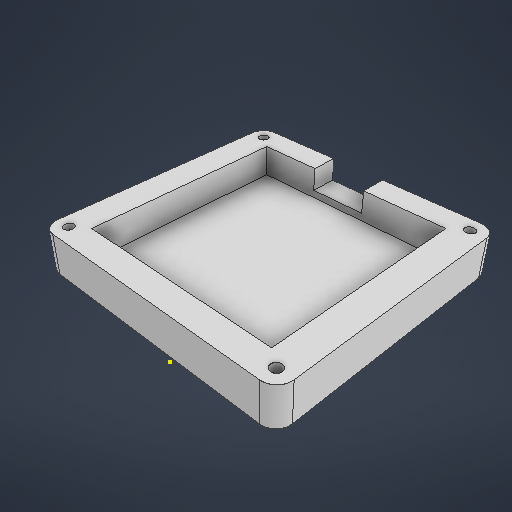
# Autodesk Inventor part: Case_Bottom
Saved by Autodesk Inventor 2026.1 (Build 301233000, 233)
## iProperties
Created: 2025-12-06
Part Number: Case_Bottom
Material: Generic
Document SubType Name: Modeling
Designer: chest
Density: 1 g/cm^3
Appearance: Default
Author: chest
Autodesk Inventor part; units mm, degrees
ref_plane "YZ Plane" through (0, 0, 0) normal (1, 0, 0) x (0, 1, 0)
ref_plane "XZ Plane" through (0, 0, 0) normal (0, 1, 0) x (-1, 0, 0)
ref_plane "XY Plane" through (0, 0, 0) normal (0, 0, 1) x (1, 0, 0)
sketch "Sketch1" plane through (0, 0, 0) normal (0, 1, 0) x (-1, 0, 0)
  line L0 (54.6183, -19.0153) -> (-12.4217, -19.0153)
  line L1 (-12.4217, -19.0153) -> (-12.4217, -83.5153)
  line L2 (-12.4217, -83.5153) -> (54.6183, -83.5153)
  line L3 (54.6183, -83.5153) -> (54.6183, -19.0153)
  line L4 (-21.9217, -9.5153) -> (64.1183, -9.5153)
  line L5 (64.1183, -9.5153) -> (64.1183, -93.0153)
  line L6 (64.1183, -93.0153) -> (-21.9217, -93.0153)
  line L7 (-21.9217, -93.0153) -> (-21.9217, -9.5153)
  circle A0 centre (-16.9217, -14.5153) radius 1.7
  circle A1 centre (-16.9217, -88.0153) radius 1.7
  circle A2 centre (59.1183, -88.0153) radius 1.7
  circle A3 centre (59.1183, -14.5153) radius 1.7
  circle A4 centre (59.1183, -14.5153) radius 3
  circle A5 centre (-16.9217, -14.5153) radius 3
  circle A6 centre (-16.9217, -88.0153) radius 3
  circle A7 centre (59.1183, -88.0153) radius 3
  point P0 (0, 0)
  point P1 (64.1183, -51.2653)
  dimension "d0" = 67.04
  dimension "d1" = 64.5
  dimension "d2" = 86.04
  dimension "d3" = 83.5
  dimension "d4" = 9.5
  dimension "d5" = 9.5
  dimension "d6" = 3.4
  dimension "d7" = 5
  dimension "d8" = 5
  dimension "d9" = 3.4
  dimension "d10" = 5
  dimension "d11" = 5
  dimension "d12" = 3.4
  dimension "d13" = 5
  dimension "d14" = 5
  dimension "d15" = 3.4
  dimension "d16" = 5
  dimension "d17" = 5
  dimension "d18" = 6
  dimension "d19" = 6
  dimension "d20" = 6
  dimension "d21" = 6
  constraints: 16 end point, 8 centre point, 4 coincident, 4 parallel, 2 horizontal, 2 perpendicular, 1 midpoint
  measures "d0" distance of L2.end L1.end
  measures "d1" distance of L1.end L0.end
  measures "d2" distance of L5.end L6.end
  measures "d3" distance of L4.end L5.end
  measures "d4" distance between parallel lines of L6 L2
  measures "d5" distance from line of point (64.118, -51.265) L3
  measures "d6" diameter of A0
  measures "d7" distance from line of L4 A0.centre
  measures "d8" distance from line of L7 A0.centre
  measures "d9" diameter of A1
  measures "d10" distance from line of L7 A1.centre
  measures "d11" distance from line of L6 A1.centre
  measures "d12" diameter of A2
  measures "d13" distance from line of L6 A2.centre
  measures "d14" distance from line of L5 A2.centre
  measures "d15" diameter of A3
  measures "d16" distance from line of L5 A3.centre
  measures "d17" distance from line of L4 A3.centre
  measures "d18" diameter of A4
  measures "d19" diameter of A5
  measures "d20" diameter of A6
  measures "d21" diameter of A7
extrude "Extrusion1" add sketch "Sketch1" along normal blind 13 contours L3 L2 L1 L0 | L4 L5 L6 L7 | A0 | A1 | A2 | A3 | A4 | A5 | A6 | A7
sketch "Sketch3" plane through (0, 13, 0) normal (0, 1, 0) x (1, 0, 0)
  circle A0 centre (-59.1183, 14.5153) radius 1.7
  line L0 (-64.1183, 9.5153) -> (21.9217, 9.5153) projected
  line L1 (-64.1183, 93.0153) -> (-64.1183, 9.5153) projected
  circle A1 centre (16.9217, 14.5153) radius 1.7
  line L2 (21.9217, 9.5153) -> (21.9217, 93.0153) projected
  circle A2 centre (16.9217, 88.0153) radius 1.7
  line L3 (21.9217, 93.0153) -> (-64.1183, 93.0153) projected
  circle A3 centre (-59.1183, 88.0153) radius 1.7
  point P0 (0, 0)
  dimension "d24" = 3.4
  dimension "d25" = 5
  dimension "d26" = 5
  dimension "d27" = 3.4
  dimension "d28" = 5
  dimension "d29" = 5
  dimension "d30" = 3.4
  dimension "d31" = 5
  dimension "d32" = 5
  dimension "d33" = 3.4
  dimension "d34" = 5
  dimension "d35" = 5
  constraints: 4 centre point
  measures "d24" diameter of A0
  measures "d25" distance from line of L0 A0.centre
  measures "d26" distance from line of A0.centre L1
  measures "d27" diameter of A1
  measures "d28" distance from line of L0 A1.centre
  measures "d29" distance from line of L2 A1.centre
  measures "d30" diameter of A2
  measures "d31" distance from line of L3 A2.centre
  measures "d32" distance from line of L2 A2.centre
  measures "d33" diameter of A3
  measures "d34" distance from line of L3 A3.centre
  measures "d35" distance from line of L1 A3.centre
extrude "Extrusion2" cut sketch "Sketch3" against normal blind 13 contours A0 | A1 | A2 | A3
sketch "Sketch6" plane through (0, 13, 0) normal (0, 1, 0) x (1, 0, 0)
  point P0 (0, 0)
sketch "Sketch7" plane through (0, 13, 0) normal (0, 1, 0) x (1, 0, 0)
  line L0 (21.9217, 93.0153) -> (-64.1183, 93.0153) projected
  line L1 (-54.1183, 84.2853) -> (11.9217, 84.2853)
  line L2 (21.9217, 9.5153) -> (21.9217, 93.0153) projected
  line L3 (-64.1183, 9.5153) -> (21.9217, 9.5153) projected
  line L4 (-21.0983, 18.2453) -> (-54.1183, 18.2453)
  line L5 (-21.0983, 18.2453) -> (11.9217, 18.2453)
  line L6 (-54.1183, 84.2853) -> (-54.1183, 18.2453)
  line L7 (11.9217, 18.2453) -> (11.9217, 84.2853)
  point P0 (0, 0)
  constraints: 10 end point, 1 parallel, 1 vertical
extrude "Extrusion3" cut sketch "Sketch7" against normal blind 10
fillet "Fillet1" radius 5 4 edges at (-64.1183, 6.5, -9.5153) (21.9217, 6.5, -9.5153) (21.9217, 6.5, -93.0153) (-64.1183, 6.5, -93.0153)
sketch "Sketch8" plane through (0, 13, 0) normal (0, 1, 0) x (1, 0, 0)
  line L0 (-54.1183, 84.2853) -> (11.9217, 84.2853) projected
  line L1 (16.9217, 93.0153) -> (-59.1183, 93.0153) projected
  line L2 (-34.1183, 84.2853) -> (-15.6183, 84.2853)
  line L3 (-15.6183, 84.2853) -> (-15.6183, 93.0153)
  line L4 (-15.6183, 93.0153) -> (-34.1183, 93.0153)
  line L5 (-34.1183, 93.0153) -> (-34.1183, 84.2853)
  line L6 (-64.1183, 88.0153) -> (-64.1183, 14.5153) projected
  point P0 (0, 0)
  dimension "d48" = 18.5
  dimension "d49" = 30
  constraints: 8 end point, 2 parallel, 2 point on line, 1 horizontal, 1 perpendicular
  measures "d48" distance of L4.end L3.end
  measures "d49" distance between parallel lines of L6 L5
extrude "Extrusion4" cut sketch "Sketch8" against normal blind 7.5
sketch "Sketch9" plane through (0, 0, 0) normal (0, -1, 0) x (1, 0, 0)
  line L0 (11.89, -89.9498) -> (-24.6442, -89.9498) construction
  line L1 (-24.6442, -89.9498) -> (-24.6442, -85.133) construction
  line L2 (-24.6442, -85.133) -> (11.89, -85.133) construction
  line L3 (11.89, -85.133) -> (11.89, -89.9498) construction
  spline S0 degree 2 poles (9.1235, -86.3163) (9.4199, -86.3163) (9.9213, -86.5164) (10.1041, -86.7164) knots 0 0 0 1 2 2 2
  spline S1 degree 2 poles (10.1041, -86.7164) (10.2869, -86.914) (10.4869, -87.5068) (10.4869, -87.8922) knots 0 0 0 1 2 2 2
  spline S2 degree 2 poles (10.4869, -87.8922) (10.4869, -88.275) (10.2918, -88.8431) (10.1066, -89.0531) knots 0 0 0 1 2 2 2
  spline S3 degree 2 poles (10.1066, -89.0531) (9.9238, -89.2581) (9.4248, -89.473) (9.1161, -89.473) knots 0 0 0 1 2 2 2
  spline S4 degree 2 poles (9.1161, -89.473) (8.9629, -89.473) (8.6937, -89.4285) (8.5801, -89.3939) knots 0 0 0 1 2 2 2
  spline S5 degree 2 poles (8.5801, -89.3939) (8.4813, -89.3618) (8.2763, -89.2704) (8.175, -89.2161) knots 0 0 0 1 2 2 2
  line L4 (8.175, -89.2161) -> (8.175, -88.727)
  line L5 (8.175, -88.727) -> (8.2071, -88.727)
  spline S6 degree 2 poles (8.2071, -88.727) (8.2615, -88.7764) (8.4294, -88.9147) (8.5504, -88.9814) knots 0 0 0 1 2 2 2
  spline S7 degree 2 poles (8.5504, -88.9814) (8.6665, -89.0457) (8.9407, -89.1272) (9.1186, -89.1272) knots 0 0 0 1 2 2 2
  spline S8 degree 2 poles (9.1186, -89.1272) (9.3137, -89.1272) (9.662, -88.9666) (9.7929, -88.8135) knots 0 0 0 1 2 2 2
  spline S9 degree 2 poles (9.7929, -88.8135) (9.9213, -88.6579) (10.0646, -88.1861) (10.0646, -87.8922) knots 0 0 0 1 2 2 2
  spline S10 degree 2 poles (10.0646, -87.8922) (10.0646, -87.5785) (9.9139, -87.1265) (9.783, -86.9708) knots 0 0 0 1 2 2 2
  spline S11 degree 2 poles (9.783, -86.9708) (9.6545, -86.8202) (9.3112, -86.667) (9.1186, -86.667) knots 0 0 0 1 2 2 2
  spline S12 degree 2 poles (9.1186, -86.667) (8.9432, -86.667) (8.6443, -86.7535) (8.5282, -86.8177) knots 0 0 0 1 2 2 2
  spline S13 degree 2 poles (8.5282, -86.8177) (8.4171, -86.8819) (8.2516, -87.0153) (8.2046, -87.0622) knots 0 0 0 1 2 2 2
  line L6 (8.2046, -87.0622) -> (8.175, -87.0622)
  line L7 (8.175, -87.0622) -> (8.175, -86.5781)
  spline S14 degree 2 poles (8.175, -86.5781) (8.2763, -86.5312) (8.4541, -86.4447) (8.5801, -86.4052) knots 0 0 0 1 2 2 2
  spline S15 degree 2 poles (8.5801, -86.4052) (8.7135, -86.3608) (8.9407, -86.3163) (9.1235, -86.3163) knots 0 0 0 1 2 2 2
  line L8 (6.031, -86.3706) -> (6.4164, -86.3706)
  line L9 (6.4164, -86.3706) -> (6.4164, -87.6748)
  spline S16 degree 2 poles (6.4164, -87.6748) (6.4164, -87.8329) (6.446, -88.1046) (6.4905, -88.1861) knots 0 0 0 1 2 2 2
  spline S17 degree 2 poles (6.4905, -88.1861) (6.5374, -88.2725) (6.7053, -88.3565) (6.8486, -88.3565) knots 0 0 0 1 2 2 2
  spline S18 degree 2 poles (6.8486, -88.3565) (6.9919, -88.3565) (7.2957, -88.2034) (7.4414, -88.0799) knots 0 0 0 1 2 2 2
  line L10 (7.4414, -88.0799) -> (7.4414, -86.3706)
  line L11 (7.4414, -86.3706) -> (7.8267, -86.3706)
  line L12 (7.8267, -86.3706) -> (7.8267, -89.5545)
  line L13 (7.8267, -89.5545) -> (7.4414, -89.5545)
  line L14 (7.4414, -89.5545) -> (7.4414, -88.4035)
  spline S19 degree 2 poles (7.4414, -88.4035) (7.2685, -88.5591) (6.9351, -88.7221) (6.7473, -88.7221) knots 0 0 0 1 2 2 2
  spline S20 degree 2 poles (6.7473, -88.7221) (6.4114, -88.7221) (6.031, -88.2775) (6.031, -87.8551) knots 0 0 0 1 2 2 2
  line L15 (6.031, -87.8551) -> (6.031, -86.3706)
  spline S21 degree 2 poles (4.4971, -86.3188) (5.0455, -86.3188) (5.6482, -86.9338) (5.6482, -87.5019) knots 0 0 0 1 2 2 2
  spline S22 degree 2 poles (5.6482, -87.5019) (5.6482, -88.0601) (5.0628, -88.7221) (4.591, -88.7221) knots 0 0 0 1 2 2 2
  spline S23 degree 2 poles (4.591, -88.7221) (4.3786, -88.7221) (4.0501, -88.5986) (3.929, -88.4677) knots 0 0 0 1 2 2 2
  spline S24 degree 2 poles (3.929, -88.4677) (3.8055, -88.3368) (3.6746, -87.9589) (3.6746, -87.6847) knots 0 0 0 1 2 2 2
  line L16 (3.6746, -87.6847) -> (3.6746, -87.4747)
  line L17 (3.6746, -87.4747) -> (5.2579, -87.4747)
  spline S25 degree 2 poles (5.2579, -87.4747) (5.2579, -87.0771) (4.8578, -86.6547) (4.5021, -86.6547) knots 0 0 0 1 2 2 2
  spline S26 degree 2 poles (4.5021, -86.6547) (4.3761, -86.6547) (4.1316, -86.7115) (4.0328, -86.756) knots 0 0 0 1 2 2 2
  spline S27 degree 2 poles (4.0328, -86.756) (3.929, -86.8054) (3.7858, -86.8918) (3.7389, -86.9313) knots 0 0 0 1 2 2 2
  line L18 (3.7389, -86.9313) -> (3.7166, -86.9313)
  line L19 (3.7166, -86.9313) -> (3.7166, -86.5114)
  spline S28 degree 2 poles (3.7166, -86.5114) (3.7833, -86.4843) (3.9859, -86.4052) (4.0649, -86.383) knots 0 0 0 1 2 2 2
  spline S29 degree 2 poles (4.0649, -86.383) (4.176, -86.3509) (4.3588, -86.3188) (4.4971, -86.3188) knots 0 0 0 1 2 2 2
  spline S30 degree 2 poles (4.0501, -87.7687) (4.055, -87.9243) (4.1192, -88.1515) (4.181, -88.2281) knots 0 0 0 1 2 2 2
  spline S31 degree 2 poles (4.181, -88.2281) (4.2477, -88.3145) (4.4576, -88.4059) (4.6132, -88.4059) knots 0 0 0 1 2 2 2
  spline S32 degree 2 poles (4.6132, -88.4059) (4.7664, -88.4059) (4.9813, -88.3145) (5.0702, -88.2256) knots 0 0 0 1 2 2 2
  spline S33 degree 2 poles (5.0702, -88.2256) (5.1566, -88.1342) (5.2456, -87.9144) (5.2579, -87.7687) knots 0 0 0 1 2 2 2
  line L20 (5.2579, -87.7687) -> (4.0501, -87.7687)
  spline S34 degree 2 poles (2.6669, -86.3163) (2.8966, -86.3163) (3.2943, -86.4398) (3.4252, -86.509) knots 0 0 0 1 2 2 2
  line L21 (3.4252, -86.509) -> (3.4252, -86.9412)
  line L22 (3.4252, -86.9412) -> (3.4054, -86.9412)
  spline S35 degree 2 poles (3.4054, -86.9412) (3.356, -86.9017) (3.2226, -86.8078) (3.1115, -86.756) knots 0 0 0 1 2 2 2
  spline S36 degree 2 poles (3.1115, -86.756) (3.0151, -86.709) (2.778, -86.6399) (2.652, -86.6399) knots 0 0 0 1 2 2 2
  spline S37 degree 2 poles (2.652, -86.6399) (2.5607, -86.6399) (2.3507, -86.6819) (2.3013, -86.7164) knots 0 0 0 1 2 2 2
  spline S38 degree 2 poles (2.3013, -86.7164) (2.2297, -86.7634) (2.1655, -86.8696) (2.1655, -86.9783) knots 0 0 0 1 2 2 2
  spline S39 degree 2 poles (2.1655, -86.9783) (2.1655, -87.1141) (2.3137, -87.2549) (2.5038, -87.3018) knots 0 0 0 1 2 2 2
  spline S40 degree 2 poles (2.5038, -87.3018) (2.5779, -87.3191) (2.8151, -87.3685) (2.9163, -87.3957) knots 0 0 0 1 2 2 2
  spline S41 degree 2 poles (2.9163, -87.3957) (3.1782, -87.4723) (3.4153, -87.7884) (3.4153, -88.0132) knots 0 0 0 1 2 2 2
  spline S42 degree 2 poles (3.4153, -88.0132) (3.4153, -88.3244) (2.9484, -88.7122) (2.5631, -88.7122) knots 0 0 0 1 2 2 2
  spline S43 degree 2 poles (2.5631, -88.7122) (2.3729, -88.7122) (1.9876, -88.6183) (1.8567, -88.5467) knots 0 0 0 1 2 2 2
  line L23 (1.8567, -88.5467) -> (1.8567, -88.1342)
  line L24 (1.8567, -88.1342) -> (1.8765, -88.1342)
  spline S44 degree 2 poles (1.8765, -88.1342) (2.0247, -88.2528) (2.3853, -88.3886) (2.5705, -88.3886) knots 0 0 0 1 2 2 2
  spline S45 degree 2 poles (2.5705, -88.3886) (2.7607, -88.3886) (3.0226, -88.2281) (3.0226, -88.0675) knots 0 0 0 1 2 2 2
  spline S46 degree 2 poles (3.0226, -88.0675) (3.0226, -87.9218) (2.8669, -87.781) (2.694, -87.7366) knots 0 0 0 1 2 2 2
  spline S47 degree 2 poles (2.694, -87.7366) (2.6101, -87.7143) (2.3976, -87.6699) (2.2815, -87.6427) knots 0 0 0 1 2 2 2
  spline S48 degree 2 poles (2.2815, -87.6427) (2.0296, -87.5785) (1.7727, -87.2845) (1.7727, -87.0301) knots 0 0 0 1 2 2 2
  spline S49 degree 2 poles (1.7727, -87.0301) (1.7727, -86.8819) (1.8888, -86.6201) (2.0024, -86.5238) knots 0 0 0 1 2 2 2
  spline S50 degree 2 poles (2.0024, -86.5238) (2.1235, -86.4225) (2.4322, -86.3163) (2.6669, -86.3163) knots 0 0 0 1 2 2 2
  spline S51 degree 2 poles (0.723, -86.3262) (1.0367, -86.3262) (1.3899, -86.6843) (1.3899, -87.0721) knots 0 0 0 1 2 2 2
  line L25 (1.3899, -87.0721) -> (1.3899, -88.3392)
  line L26 (1.3899, -88.3392) -> (1.6492, -88.3392)
  line L27 (1.6492, -88.3392) -> (1.6492, -88.6579)
  line L28 (1.6492, -88.6579) -> (1.3899, -88.6579)
  line L29 (1.3899, -88.6579) -> (1.3899, -89.3149)
  line L30 (1.3899, -89.3149) -> (1.0045, -89.3149)
  line L31 (1.0045, -89.3149) -> (1.0045, -88.6579)
  line L32 (1.0045, -88.6579) -> (0.2957, -88.6579)
  line L33 (0.2957, -88.6579) -> (0.2957, -88.3392)
  line L34 (0.2957, -88.3392) -> (1.0045, -88.3392)
  line L35 (1.0045, -88.3392) -> (1.0045, -87.25)
  spline S52 degree 2 poles (1.0045, -87.25) (1.0045, -87.0771) (0.9922, -86.8869) (0.9502, -86.8054) knots 0 0 0 1 2 2 2
  spline S53 degree 2 poles (0.9502, -86.8054) (0.9156, -86.7337) (0.76, -86.6621) (0.6266, -86.6621) knots 0 0 0 1 2 2 2
  spline S54 degree 2 poles (0.6266, -86.6621) (0.5328, -86.6621) (0.3574, -86.7189) (0.3179, -86.7362) knots 0 0 0 1 2 2 2
  line L36 (0.3179, -86.7362) -> (0.2957, -86.7362)
  line L37 (0.2957, -86.7362) -> (0.2957, -86.3904)
  spline S55 degree 2 poles (0.2957, -86.3904) (0.4043, -86.3608) (0.6266, -86.3262) (0.723, -86.3262) knots 0 0 0 1 2 2 2
  spline S56 degree 2 poles (-0.9813, -86.3188) (-0.433, -86.3188) (0.1697, -86.9338) (0.1697, -87.5019) knots 0 0 0 1 2 2 2
  spline S57 degree 2 poles (0.1697, -87.5019) (0.1697, -88.0601) (-0.4157, -88.7221) (-0.8875, -88.7221) knots 0 0 0 1 2 2 2
  spline S58 degree 2 poles (-0.8875, -88.7221) (-1.0999, -88.7221) (-1.4284, -88.5986) (-1.5494, -88.4677) knots 0 0 0 1 2 2 2
  spline S59 degree 2 poles (-1.5494, -88.4677) (-1.673, -88.3368) (-1.8039, -87.9589) (-1.8039, -87.6847) knots 0 0 0 1 2 2 2
  line L38 (-1.8039, -87.6847) -> (-1.8039, -87.4747)
  line L39 (-1.8039, -87.4747) -> (-0.2206, -87.4747)
  spline S60 degree 2 poles (-0.2206, -87.4747) (-0.2206, -87.0771) (-0.6207, -86.6547) (-0.9764, -86.6547) knots 0 0 0 1 2 2 2
  spline S61 degree 2 poles (-0.9764, -86.6547) (-1.1024, -86.6547) (-1.3469, -86.7115) (-1.4457, -86.756) knots 0 0 0 1 2 2 2
  spline S62 degree 2 poles (-1.4457, -86.756) (-1.5494, -86.8054) (-1.6927, -86.8918) (-1.7396, -86.9313) knots 0 0 0 1 2 2 2
  line L40 (-1.7396, -86.9313) -> (-1.7619, -86.9313)
  line L41 (-1.7619, -86.9313) -> (-1.7619, -86.5114)
  spline S63 degree 2 poles (-1.7619, -86.5114) (-1.6952, -86.4843) (-1.4926, -86.4052) (-1.4136, -86.383) knots 0 0 0 1 2 2 2
  spline S64 degree 2 poles (-1.4136, -86.383) (-1.3024, -86.3509) (-1.1197, -86.3188) (-0.9813, -86.3188) knots 0 0 0 1 2 2 2
  spline S65 degree 2 poles (-1.4284, -87.7687) (-1.4235, -87.9243) (-1.3593, -88.1515) (-1.2975, -88.2281) knots 0 0 0 1 2 2 2
  spline S66 degree 2 poles (-1.2975, -88.2281) (-1.2308, -88.3145) (-1.0209, -88.4059) (-0.8653, -88.4059) knots 0 0 0 1 2 2 2
  spline S67 degree 2 poles (-0.8653, -88.4059) (-0.7121, -88.4059) (-0.4972, -88.3145) (-0.4083, -88.2256) knots 0 0 0 1 2 2 2
  spline S68 degree 2 poles (-0.4083, -88.2256) (-0.3219, -88.1342) (-0.2329, -87.9144) (-0.2206, -87.7687) knots 0 0 0 1 2 2 2
  line L42 (-0.2206, -87.7687) -> (-1.4284, -87.7687)
  line L43 (-3.4069, -88.2454) -> (-3.3871, -88.2454)
  spline S69 degree 2 poles (-3.3871, -88.2454) (-3.3427, -88.2577) (-3.2464, -88.2627) (-3.1797, -88.2627) knots 0 0 0 1 2 2 2
  spline S70 degree 2 poles (-3.1797, -88.2627) (-3.024, -88.2627) (-2.7178, -88.1268) (-2.5794, -87.9934) knots 0 0 0 1 2 2 2
  line L44 (-2.5794, -87.9934) -> (-2.5794, -86.3706)
  line L45 (-2.5794, -86.3706) -> (-2.1941, -86.3706)
  line L46 (-2.1941, -86.3706) -> (-2.1941, -88.6579)
  line L47 (-2.1941, -88.6579) -> (-2.5794, -88.6579)
  line L48 (-2.5794, -88.6579) -> (-2.5794, -88.317)
  spline S71 degree 2 poles (-2.5794, -88.317) (-2.7894, -88.5047) (-3.1031, -88.6579) (-3.2513, -88.6579) knots 0 0 0 1 2 2 2
  spline S72 degree 2 poles (-3.2513, -88.6579) (-3.3106, -88.6579) (-3.3699, -88.6529) (-3.4069, -88.6455) knots 0 0 0 1 2 2 2
  line L49 (-3.4069, -88.6455) -> (-3.4069, -88.2454)
  line L50 (-4.096, -89.5545) -> (-4.0071, -88.3689)
  line L51 (-4.0071, -88.3689) -> (-3.7305, -88.3689)
  line L52 (-3.7305, -88.3689) -> (-3.6416, -89.5545)
  line L53 (-3.6416, -89.5545) -> (-4.096, -89.5545)
  spline S73 degree 2 poles (-5.2075, -86.3163) (-4.9778, -86.3163) (-4.5802, -86.4398) (-4.4492, -86.509) knots 0 0 0 1 2 2 2
  line L54 (-4.4492, -86.509) -> (-4.4492, -86.9412)
  line L55 (-4.4492, -86.9412) -> (-4.469, -86.9412)
  spline S74 degree 2 poles (-4.469, -86.9412) (-4.5184, -86.9017) (-4.6518, -86.8078) (-4.7629, -86.756) knots 0 0 0 1 2 2 2
  spline S75 degree 2 poles (-4.7629, -86.756) (-4.8593, -86.709) (-5.0964, -86.6399) (-5.2224, -86.6399) knots 0 0 0 1 2 2 2
  spline S76 degree 2 poles (-5.2224, -86.6399) (-5.3138, -86.6399) (-5.5237, -86.6819) (-5.5731, -86.7164) knots 0 0 0 1 2 2 2
  spline S77 degree 2 poles (-5.5731, -86.7164) (-5.6447, -86.7634) (-5.709, -86.8696) (-5.709, -86.9783) knots 0 0 0 1 2 2 2
  spline S78 degree 2 poles (-5.709, -86.9783) (-5.709, -87.1141) (-5.5608, -87.2549) (-5.3706, -87.3018) knots 0 0 0 1 2 2 2
  spline S79 degree 2 poles (-5.3706, -87.3018) (-5.2965, -87.3191) (-5.0593, -87.3685) (-4.9581, -87.3957) knots 0 0 0 1 2 2 2
  spline S80 degree 2 poles (-4.9581, -87.3957) (-4.6963, -87.4723) (-4.4591, -87.7884) (-4.4591, -88.0132) knots 0 0 0 1 2 2 2
  spline S81 degree 2 poles (-4.4591, -88.0132) (-4.4591, -88.3244) (-4.926, -88.7122) (-5.3113, -88.7122) knots 0 0 0 1 2 2 2
  spline S82 degree 2 poles (-5.3113, -88.7122) (-5.5015, -88.7122) (-5.8868, -88.6183) (-6.0177, -88.5467) knots 0 0 0 1 2 2 2
  line L56 (-6.0177, -88.5467) -> (-6.0177, -88.1342)
  line L57 (-6.0177, -88.1342) -> (-5.9979, -88.1342)
  spline S83 degree 2 poles (-5.9979, -88.1342) (-5.8497, -88.2528) (-5.4891, -88.3886) (-5.3039, -88.3886) knots 0 0 0 1 2 2 2
  spline S84 degree 2 poles (-5.3039, -88.3886) (-5.1137, -88.3886) (-4.8519, -88.2281) (-4.8519, -88.0675) knots 0 0 0 1 2 2 2
  spline S85 degree 2 poles (-4.8519, -88.0675) (-4.8519, -87.9218) (-5.0075, -87.781) (-5.1804, -87.7366) knots 0 0 0 1 2 2 2
  spline S86 degree 2 poles (-5.1804, -87.7366) (-5.2644, -87.7143) (-5.4768, -87.6699) (-5.5929, -87.6427) knots 0 0 0 1 2 2 2
  spline S87 degree 2 poles (-5.5929, -87.6427) (-5.8448, -87.5785) (-6.1017, -87.2845) (-6.1017, -87.0301) knots 0 0 0 1 2 2 2
  spline S88 degree 2 poles (-6.1017, -87.0301) (-6.1017, -86.8819) (-5.9856, -86.6201) (-5.872, -86.5238) knots 0 0 0 1 2 2 2
  spline S89 degree 2 poles (-5.872, -86.5238) (-5.7509, -86.4225) (-5.4422, -86.3163) (-5.2075, -86.3163) knots 0 0 0 1 2 2 2
  line L58 (-10.0117, -86.3706) -> (-9.6066, -86.3706)
  line L59 (-9.6066, -86.3706) -> (-9.6066, -87.8625)
  line L60 (-9.6066, -87.8625) -> (-8.2037, -87.8625)
  line L61 (-8.2037, -87.8625) -> (-8.2037, -86.3706)
  line L62 (-8.2037, -86.3706) -> (-7.7986, -86.3706)
  line L63 (-7.7986, -86.3706) -> (-7.7986, -89.4186)
  line L64 (-7.7986, -89.4186) -> (-8.2037, -89.4186)
  line L65 (-8.2037, -89.4186) -> (-8.2037, -88.2231)
  line L66 (-8.2037, -88.2231) -> (-9.6066, -88.2231)
  line L67 (-9.6066, -88.2231) -> (-9.6066, -89.4186)
  line L68 (-9.6066, -89.4186) -> (-10.0117, -89.4186)
  line L69 (-10.0117, -89.4186) -> (-10.0117, -86.3706)
  spline S90 degree 2 poles (-11.8741, -86.6127) (-11.8272, -86.5781) (-11.6691, -86.4546) (-11.595, -86.4176) knots 0 0 0 1 2 2 2
  spline S91 degree 2 poles (-11.595, -86.4176) (-11.4937, -86.3632) (-11.3035, -86.3064) (-11.1306, -86.3064) knots 0 0 0 1 2 2 2
  spline S92 degree 2 poles (-11.1306, -86.3064) (-10.9899, -86.3064) (-10.7354, -86.4126) (-10.6391, -86.509) knots 0 0 0 1 2 2 2
  spline S93 degree 2 poles (-10.6391, -86.509) (-10.5477, -86.6028) (-10.4366, -86.8795) (-10.4366, -87.0326) knots 0 0 0 1 2 2 2
  spline S94 degree 2 poles (-10.4366, -87.0326) (-10.4366, -87.2697) (-10.6366, -87.6056) (-10.854, -87.702) knots 0 0 0 1 2 2 2
  spline S95 degree 2 poles (-10.854, -87.702) (-11.0467, -87.7909) (-11.5703, -87.8576) (-11.8741, -87.8749) knots 0 0 0 1 2 2 2
  line L70 (-11.8741, -87.8749) -> (-11.8741, -87.949)
  spline S96 degree 2 poles (-11.8741, -87.949) (-11.8741, -88.0824) (-11.7926, -88.2478) (-11.7185, -88.2948) knots 0 0 0 1 2 2 2
  spline S97 degree 2 poles (-11.7185, -88.2948) (-11.6444, -88.3417) (-11.432, -88.3713) (-11.3184, -88.3713) knots 0 0 0 1 2 2 2
  spline S98 degree 2 poles (-11.3184, -88.3713) (-11.185, -88.3713) (-10.8244, -88.2923) (-10.644, -88.2157) knots 0 0 0 1 2 2 2
  line L71 (-10.644, -88.2157) -> (-10.6218, -88.2157)
  line L72 (-10.6218, -88.2157) -> (-10.6218, -88.6085)
  spline S99 degree 2 poles (-10.6218, -88.6085) (-10.728, -88.6381) (-11.1257, -88.7122) (-11.3208, -88.7122) knots 0 0 0 1 2 2 2
  spline S100 degree 2 poles (-11.3208, -88.7122) (-11.558, -88.7122) (-11.8815, -88.6381) (-12.01, -88.5418) knots 0 0 0 1 2 2 2
  spline S101 degree 2 poles (-12.01, -88.5418) (-12.1359, -88.4479) (-12.2594, -88.149) (-12.2594, -87.9342) knots 0 0 0 1 2 2 2
  line L73 (-12.2594, -87.9342) -> (-12.2594, -86.3706)
  line L74 (-12.2594, -86.3706) -> (-11.8741, -86.3706)
  line L75 (-11.8741, -86.3706) -> (-11.8741, -86.6127)
  line L76 (-11.8741, -86.9338) -> (-11.8741, -87.5686)
  spline S102 degree 2 poles (-11.8741, -87.5686) (-11.7358, -87.5562) (-11.3184, -87.5143) (-11.1875, -87.4747) knots 0 0 0 1 2 2 2
  spline S103 degree 2 poles (-11.1875, -87.4747) (-11.0343, -87.4278) (-10.8342, -87.2327) (-10.8342, -87.0598) knots 0 0 0 1 2 2 2
  spline S104 degree 2 poles (-10.8342, -87.0598) (-10.8342, -86.8622) (-11.0565, -86.6621) (-11.269, -86.6621) knots 0 0 0 1 2 2 2
  spline S105 degree 2 poles (-11.269, -86.6621) (-11.4493, -86.6621) (-11.7457, -86.8177) (-11.8741, -86.9338) knots 0 0 0 1 2 2 2
  spline S106 degree 2 poles (-13.7093, -86.3188) (-13.4722, -86.3188) (-13.0795, -86.4645) (-12.9387, -86.6127) knots 0 0 0 1 2 2 2
  spline S107 degree 2 poles (-12.9387, -86.6127) (-12.7979, -86.7584) (-12.6423, -87.208) (-12.6423, -87.5093) knots 0 0 0 1 2 2 2
  spline S108 degree 2 poles (-12.6423, -87.5093) (-12.6423, -87.8107) (-12.8028, -88.2503) (-12.9387, -88.3985) knots 0 0 0 1 2 2 2
  spline S109 degree 2 poles (-12.9387, -88.3985) (-13.0745, -88.5492) (-13.4772, -88.7097) (-13.7093, -88.7097) knots 0 0 0 1 2 2 2
  spline S110 degree 2 poles (-13.7093, -88.7097) (-13.8971, -88.7097) (-14.2478, -88.6035) (-14.3837, -88.5344) knots 0 0 0 1 2 2 2
  line L77 (-14.3837, -88.5344) -> (-14.3837, -88.1021)
  line L78 (-14.3837, -88.1021) -> (-14.3614, -88.1021)
  spline S111 degree 2 poles (-14.3614, -88.1021) (-14.3194, -88.1367) (-14.191, -88.2256) (-14.0996, -88.2725) knots 0 0 0 1 2 2 2
  spline S112 degree 2 poles (-14.0996, -88.2725) (-14.0181, -88.3121) (-13.8007, -88.3738) (-13.7019, -88.3738) knots 0 0 0 1 2 2 2
  spline S113 degree 2 poles (-13.7019, -88.3738) (-13.4031, -88.3738) (-13.04, -87.9218) (-13.04, -87.5093) knots 0 0 0 1 2 2 2
  spline S114 degree 2 poles (-13.04, -87.5093) (-13.04, -87.1067) (-13.3907, -86.6547) (-13.7019, -86.6547) knots 0 0 0 1 2 2 2
  spline S115 degree 2 poles (-13.7019, -86.6547) (-13.8897, -86.6547) (-14.2305, -86.8103) (-14.3614, -86.9313) knots 0 0 0 1 2 2 2
  line L79 (-14.3614, -86.9313) -> (-14.3837, -86.9313)
  line L80 (-14.3837, -86.9313) -> (-14.3837, -86.4991)
  spline S116 degree 2 poles (-14.3837, -86.4991) (-14.3268, -86.4719) (-14.1539, -86.3953) (-14.0848, -86.378) knots 0 0 0 1 2 2 2
  spline S117 degree 2 poles (-14.0848, -86.378) (-13.986, -86.3484) (-13.8304, -86.3188) (-13.7093, -86.3188) knots 0 0 0 1 2 2 2
  line L81 (-16.6289, -86.3706) -> (-16.1225, -86.3706)
  line L82 (-16.1225, -86.3706) -> (-15.2729, -87.4747)
  line L83 (-15.2729, -87.4747) -> (-15.1197, -87.3265)
  line L84 (-15.1197, -87.3265) -> (-15.1197, -86.3706)
  line L85 (-15.1197, -86.3706) -> (-14.7344, -86.3706)
  line L86 (-14.7344, -86.3706) -> (-14.7344, -89.5545)
  line L87 (-14.7344, -89.5545) -> (-15.1197, -89.5545)
  line L88 (-15.1197, -89.5545) -> (-15.1197, -87.6921)
  line L89 (-15.1197, -87.6921) -> (-16.0237, -88.6579)
  line L90 (-16.0237, -88.6579) -> (-16.5029, -88.6579)
  line L91 (-16.5029, -88.6579) -> (-15.5643, -87.702)
  line L92 (-15.5643, -87.702) -> (-16.6289, -86.3706)
  spline S118 degree 2 poles (-18.7383, -87.576) (-18.7383, -87.003) (-18.1924, -86.3262) (-17.775, -86.3262) knots 0 0 0 1 2 2 2
  spline S119 degree 2 poles (-17.775, -86.3262) (-17.6046, -86.3262) (-17.3427, -86.4052) (-17.2069, -86.4867) knots 0 0 0 1 2 2 2
  line L93 (-17.2069, -86.4867) -> (-17.2069, -85.5284)
  line L94 (-17.2069, -85.5284) -> (-16.8216, -85.5284)
  line L95 (-16.8216, -85.5284) -> (-16.8216, -88.6579)
  line L96 (-16.8216, -88.6579) -> (-17.2069, -88.6579)
  line L97 (-17.2069, -88.6579) -> (-17.2069, -88.4183)
  spline S120 degree 2 poles (-17.2069, -88.4183) (-17.3501, -88.5492) (-17.7009, -88.7221) (-17.9059, -88.7221) knots 0 0 0 1 2 2 2
  spline S121 degree 2 poles (-17.9059, -88.7221) (-18.2986, -88.7221) (-18.7383, -88.0996) (-18.7383, -87.576) knots 0 0 0 1 2 2 2
  spline S122 degree 2 poles (-18.3406, -87.5315) (-18.3406, -87.9243) (-18.0911, -88.3565) (-17.812, -88.3565) knots 0 0 0 1 2 2 2
  spline S123 degree 2 poles (-17.812, -88.3565) (-17.649, -88.3565) (-17.3427, -88.2108) (-17.2069, -88.0972) knots 0 0 0 1 2 2 2
  line L98 (-17.2069, -88.0972) -> (-17.2069, -86.7979)
  spline S124 degree 2 poles (-17.2069, -86.7979) (-17.3576, -86.7263) (-17.5724, -86.672) (-17.7108, -86.672) knots 0 0 0 1 2 2 2
  spline S125 degree 2 poles (-17.7108, -86.672) (-18.0096, -86.672) (-18.3406, -87.1116) (-18.3406, -87.5315) knots 0 0 0 1 2 2 2
  spline S126 degree 2 poles (-20.413, -86.6127) (-20.366, -86.5781) (-20.208, -86.4546) (-20.1339, -86.4176) knots 0 0 0 1 2 2 2
  spline S127 degree 2 poles (-20.1339, -86.4176) (-20.0326, -86.3632) (-19.8424, -86.3064) (-19.6695, -86.3064) knots 0 0 0 1 2 2 2
  spline S128 degree 2 poles (-19.6695, -86.3064) (-19.5287, -86.3064) (-19.2743, -86.4126) (-19.178, -86.509) knots 0 0 0 1 2 2 2
  spline S129 degree 2 poles (-19.178, -86.509) (-19.0866, -86.6028) (-18.9754, -86.8795) (-18.9754, -87.0326) knots 0 0 0 1 2 2 2
  spline S130 degree 2 poles (-18.9754, -87.0326) (-18.9754, -87.2697) (-19.1755, -87.6056) (-19.3928, -87.702) knots 0 0 0 1 2 2 2
  spline S131 degree 2 poles (-19.3928, -87.702) (-19.5855, -87.7909) (-20.1092, -87.8576) (-20.413, -87.8749) knots 0 0 0 1 2 2 2
  line L99 (-20.413, -87.8749) -> (-20.413, -87.949)
  spline S132 degree 2 poles (-20.413, -87.949) (-20.413, -88.0824) (-20.3315, -88.2478) (-20.2574, -88.2948) knots 0 0 0 1 2 2 2
  spline S133 degree 2 poles (-20.2574, -88.2948) (-20.1833, -88.3417) (-19.9708, -88.3713) (-19.8572, -88.3713) knots 0 0 0 1 2 2 2
  spline S134 degree 2 poles (-19.8572, -88.3713) (-19.7238, -88.3713) (-19.3632, -88.2923) (-19.1829, -88.2157) knots 0 0 0 1 2 2 2
  line L100 (-19.1829, -88.2157) -> (-19.1607, -88.2157)
  line L101 (-19.1607, -88.2157) -> (-19.1607, -88.6085)
  spline S135 degree 2 poles (-19.1607, -88.6085) (-19.2669, -88.6381) (-19.6645, -88.7122) (-19.8597, -88.7122) knots 0 0 0 1 2 2 2
  spline S136 degree 2 poles (-19.8597, -88.7122) (-20.0968, -88.7122) (-20.4204, -88.6381) (-20.5488, -88.5418) knots 0 0 0 1 2 2 2
  spline S137 degree 2 poles (-20.5488, -88.5418) (-20.6748, -88.4479) (-20.7983, -88.149) (-20.7983, -87.9342) knots 0 0 0 1 2 2 2
  line L102 (-20.7983, -87.9342) -> (-20.7983, -86.3706)
  line L103 (-20.7983, -86.3706) -> (-20.413, -86.3706)
  line L104 (-20.413, -86.3706) -> (-20.413, -86.6127)
  line L105 (-20.413, -86.9338) -> (-20.413, -87.5686)
  spline S138 degree 2 poles (-20.413, -87.5686) (-20.2746, -87.5562) (-19.8572, -87.5143) (-19.7263, -87.4747) knots 0 0 0 1 2 2 2
  spline S139 degree 2 poles (-19.7263, -87.4747) (-19.5732, -87.4278) (-19.3731, -87.2327) (-19.3731, -87.0598) knots 0 0 0 1 2 2 2
  spline S140 degree 2 poles (-19.3731, -87.0598) (-19.3731, -86.8622) (-19.5954, -86.6621) (-19.8078, -86.6621) knots 0 0 0 1 2 2 2
  spline S141 degree 2 poles (-19.8078, -86.6621) (-19.9881, -86.6621) (-20.2845, -86.8177) (-20.413, -86.9338) knots 0 0 0 1 2 2 2
  line L106 (-23.0979, -86.3706) -> (-22.7125, -86.3706)
  line L107 (-22.7125, -86.3706) -> (-22.7125, -86.6028)
  spline S142 degree 2 poles (-22.7125, -86.6028) (-22.6236, -86.5287) (-22.4927, -86.4299) (-22.4038, -86.3879) knots 0 0 0 1 2 2 2
  spline S143 degree 2 poles (-22.4038, -86.3879) (-22.3223, -86.3484) (-22.1469, -86.3064) (-22.0308, -86.3064) knots 0 0 0 1 2 2 2
  spline S144 degree 2 poles (-22.0308, -86.3064) (-21.8431, -86.3064) (-21.5269, -86.462) (-21.4158, -86.6127) knots 0 0 0 1 2 2 2
  spline S145 degree 2 poles (-21.4158, -86.6127) (-21.3046, -86.7634) (-21.1811, -87.208) (-21.1811, -87.497) knots 0 0 0 1 2 2 2
  spline S146 degree 2 poles (-21.1811, -87.497) (-21.1811, -87.7983) (-21.3367, -88.238) (-21.4726, -88.4035) knots 0 0 0 1 2 2 2
  spline S147 degree 2 poles (-21.4726, -88.4035) (-21.5986, -88.5517) (-21.9518, -88.7221) (-22.1469, -88.7221) knots 0 0 0 1 2 2 2
  spline S148 degree 2 poles (-22.1469, -88.7221) (-22.3173, -88.7221) (-22.5718, -88.6455) (-22.7125, -88.5665) knots 0 0 0 1 2 2 2
  line L108 (-22.7125, -88.5665) -> (-22.7125, -89.5545)
  line L109 (-22.7125, -89.5545) -> (-23.0979, -89.5545)
  line L110 (-23.0979, -89.5545) -> (-23.0979, -86.3706)
  line L111 (-22.7125, -86.9264) -> (-22.7125, -88.2478)
  spline S149 degree 2 poles (-22.7125, -88.2478) (-22.5693, -88.317) (-22.342, -88.3689) (-22.2111, -88.3689) knots 0 0 0 1 2 2 2
  spline S150 degree 2 poles (-22.2111, -88.3689) (-21.9147, -88.3689) (-21.5788, -87.9243) (-21.5788, -87.5044) knots 0 0 0 1 2 2 2
  spline S151 degree 2 poles (-21.5788, -87.5044) (-21.5788, -87.0993) (-21.8357, -86.672) (-22.1197, -86.672) knots 0 0 0 1 2 2 2
  spline S152 degree 2 poles (-22.1197, -86.672) (-22.2704, -86.672) (-22.5767, -86.8103) (-22.7125, -86.9264) knots 0 0 0 1 2 2 2
  point P0 (0, 0)
  constraints: 2 other
emboss "Emboss1" sketch "Sketch9" operation cut depth 0.2 direction (0, 1, 0)
body "Solid1"
